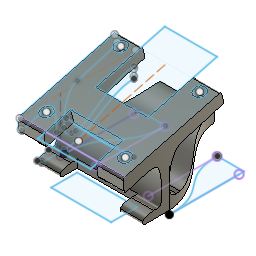
front-short (Autodesk Fusion 360 design; units mm, degrees)
Autodesk Fusion 360 part; units mm, degrees
sketch "Skizze1" plane through (0, 0, 0) normal (1, 0, 0) x (0, 1, 0)
  line L0 (-5, 1) -> (1, 1)
  line L1 (0, 0) -> (0, 14.4867) construction
  line L2 (0, 14.4867) -> (-11.359, 14.4867) construction
  line L3 (0, 14.4867) -> (20, 14.4867) construction
  line L4 (-11.0357, 11.4071) -> (-11.3143, 14.0608)
  line L5 (-10.9451, 14.5964) -> (14.3234, 21.29)
  spline S0 degree 5 poles (1, 1) (1.7814, 1) (3.3248, 1.1441) (5.5821, 1.792) (8.4987, 3.3498) (12.0892, 5.7087) (15.005, 7.2713) (17.261, 7.926) (18.8034, 8.0762) (19.5841, 8.0797) knots 0 0 0 0 0 0 0.2 0.4 0.6 0.8 1 1 1 1 1 1
  line L6 (-1, 1) -> (3, 1)
  line L7 (17.575, 8.0666) -> (21.5749, 8.0843)
  line L8 (20.0592, 10.4933) -> (20.0592, 8.5791)
  arc A0 (20.0592, 10.4933) -> (19.5271, 10.9923) centre (19.5592, 10.4933) ccw
  arc A1 (19.5841, 8.0797) -> (20.0592, 8.5791) centre (19.5592, 8.5791) ccw
  arc A2 (14.9514, 20.8065) -> (14.3234, 21.29) centre (14.4514, 20.8067) ccw
  arc A3 (-11.0357, 11.4071) -> (-10.2738, 11.0351) centre (-10.5384, 11.4593) ccw
  spline S1 degree 5 poles (-10.2738, 11.0351) (-9.3554, 11.3092) (-7.6686, 11.819) (-5.5882, 12.4682) (-3.6466, 13.0308) (-2.2683, 12.9173) (-1.5391, 11.673) (-1.1522, 9.3083) (-0.9068, 6.1018) (-1.0418, 3.5276) (-1.7721, 2.8079) (-2.4824, 3.0034) (-2.8857, 3.1016) (-3.0583, 3.0428) (-3.1208, 2.9828) knots 0 0 0 0 0 0 0.1 0.2 0.3 0.4 0.5 0.6 0.7 0.8 0.9 1 1 1 1 1 1
  line L9 (-14.6982, 9.7143) -> (-5.8494, 12.3559)
  line L10 (-1, 9) -> (-1, 3)
  line L11 (-2.4936, 3.5857) -> (-3.7479, 2.3798)
  spline S2 degree 5 poles (4.5055, 15.1733) (4.1976, 15.0836) (3.6204, 14.8401) (2.8706, 14.2825) (2.0929, 13.1886) (1.4422, 11.4286) (1.0571, 9.5179) (0.8923, 7.6993) (0.918, 6.1755) (1.144, 5.0495) (1.5922, 4.2914) (2.0891, 3.9529) (2.5177, 3.8314) (2.8242, 3.8071) (2.9826, 3.8091) knots 0 0 0 0 0 0 0.1 0.2 0.3 0.4 0.5 0.6 0.7 0.8 0.9 1 1 1 1 1 1
  spline S3 degree 5 poles (19.5271, 10.9923) (18.7621, 10.9405) (17.2555, 10.7096) (15.0658, 9.982) (12.2831, 8.4027) (9.0678, 6.0947) (6.7884, 4.5873) (5.3121, 3.9616) (4.4471, 3.8224) (4.0444, 3.8224) knots 0 0 0 0 0 0 0.2 0.4 0.6 0.8 1 1 1 1 1 1
  line L12 (21.451, 11.1225) -> (17.6033, 10.862)
  line L13 (5.0444, 3.8225) -> (3.0444, 3.8223)
  line L14 (6.7734, 15.8337) -> (2.2376, 14.5129)
  line L15 (0.6508, 8.5379) -> (1.3492, 3.4621)
  line L16 (0.5609, 3.7787) -> (5.4043, 3.8394)
  line L17 (2.9826, 3.8091) -> (4.0444, 3.8224)
  spline S4 degree 5 poles (-5, 1) (-5.1368, 0.9954) (-5.3837, 0.9989) (-5.6734, 1.0427) (-5.921, 1.1673) (-6.0765, 1.3967) (-6.1253, 1.6162) (-6.1334, 1.7945) (-6.1269, 1.9191) (-6.1208, 1.9828) knots 0 0 0 0 0 0 0.2 0.4 0.6 0.8 1 1 1 1 1 1
  spline S5 degree 5 poles (-3.1208, 2.9828) (-3.2537, 2.9767) (-3.5181, 2.9606) (-3.9103, 2.9246) (-4.4234, 2.8514) (-5.0408, 2.697) (-5.5035, 2.4916) (-5.8241, 2.2684) (-6.0241, 2.0839) (-6.1208, 1.9828) knots 0 0 0 0 0 0 0.2 0.4 0.6 0.8 1 1 1 1 1 1
  line L18 (-4.539, 1.0156) -> (-5.461, 0.9844)
  line L19 (-5.8879, 2.2266) -> (-6.3536, 1.7389)
  line L20 (4.5055, 15.1733) -> (15.1184, 18.3262)
  line L21 (15.4586, 18.9363) -> (14.9514, 20.8065)
  arc A4 (15.1184, 18.3262) -> (15.4586, 18.9363) centre (14.976, 18.8055) ccw
  arc A5 (-10.9451, 14.5964) -> (-11.3143, 14.0608) centre (-10.817, 14.113) ccw
  point P0 (-1, 6)
  point P1 (1, 6)
  dimension "d1" = 0.5
  dimension "d2" = 0.5
  dimension "d3" = 0.5
  dimension "d5" = 0.5
  dimension "d24" = 0.5
  dimension "d27" = 0.5
  constraint horizontal L0
  constraint coincident L1.start origin
  constraint perpendicular L0 L1
  constraint perpendicular L1 L2
  constraint perpendicular L1 L3
  constraint midpoint L0.end L6
  constraint vertical L8
  constraint tangent L8 A0
  constraint tangent S0 A1
  constraint tangent L8 A1
  constraint tangent L5 A2
  constraint tangent L4 A3
  constraint midpoint A3.end L9
  constraint midpoint P0 L10
  constraint midpoint S1.end L11
  constraint midpoint A0.end L12
  constraint midpoint S3.end L13
  constraint midpoint S2.start L14
  constraint midpoint P1 L15
  constraint midpoint S2.end L16
  constraint midpoint L0.start L18
  constraint midpoint S4.end L19
  constraint tangent L20 A4
  constraint tangent L21 A4
  constraint coincident L2.end L4
  constraint coincident L2.end L5
  constraint tangent L4 A5
  constraint tangent L5 A5
  measures "d1" radius of A0
  measures "d2" radius of A1
  measures "d3" radius of A2
  measures "d5" radius of A3
  measures "d24" radius of A4
  measures "d27" radius of A5
extrude "Extrusion1" add sketch "Skizze1" along normal blind 28
sketch "Skizze2" plane through (0, -4.3307, 16.3485) normal (0, -0.256068, 0.966659) x (1, 0, 0)
  line L0 (0, 19.2975) -> (0, -6.8425)
  line L1 (28, -6.8425) -> (28, 19.2975)
  line L2 (28, 19.2975) -> (0, 19.2975)
  line L3 (14, -5.0283) -> (14, 19.2975) construction
  line L4 (20.9548, 0) -> (7, 0)
  line L5 (20.9199, 7) -> (7, 7)
  line L6 (20.9199, 7) -> (20.9199, 26)
  line L7 (20.9199, 26) -> (7, 26)
  line L8 (7, 26) -> (7, 7)
  line L9 (7, 0) -> (7, -9)
  line L10 (7, -9) -> (21.0129, -9)
  line L11 (21.0129, -9) -> (20.9548, 0)
  circle A0 centre (3.5, -3) radius 1.5
  circle A1 centre (24.5, -3) radius 1.5
  line L12 (0, -6.8425) -> (28, -6.8425)
  circle A2 centre (3.5, 17.5) radius 1.5
  circle A3 centre (24.5, 17.5) radius 1.5
  dimension "d16" = 3
  dimension "d17" = 3
  dimension "d36" = 3
  dimension "d37" = 3
  constraint midpoint L2 L3.end
  constraint perpendicular L3 L4
  constraint perpendicular L2 L6
  constraint perpendicular L6 L7
  constraint perpendicular L5 L8
  constraint perpendicular L9 L10
  measures "d16" diameter of A0
  measures "d17" diameter of A1
  measures "d36" diameter of A2
  measures "d37" diameter of A3
extrude "Extrusion2" cut sketch "Skizze2" against normal blind 4.5 contours L9 L10 L11 L12 | L4 L9 L11 L12
extrude "Extrusion4" cut sketch "Skizze2" against normal blind 10 contours L2 L6 L7 L8 | L2 L5 L6 L8
sketch "Skizze3" plane through (0, 0, 0) normal (0, 0, 1) x (1, 0, 0)
  line L0 (28, 1) -> (28, 19.5841)
  line L1 (0, 1) -> (0, 19.5841)
  line L2 (7, 20.8024) -> (7, 2.4359)
  line L3 (20.9199, 2.4359) -> (20.9199, 20.8024)
  spline S0 degree 5 poles (28, 1) (28, 2.2287) (27.8554, 4.4703) (27.2053, 7.1862) (25.6424, 9.7666) (23.2775, 12.3598) (21.7146, 14.8926) (21.0645, 17.541) (20.9199, 19.7219) (20.9199, 20.9163) knots 0 0 0 0 0 0 0.2 0.4 0.6 0.8 1 1 1 1 1 1
  line L4 (28, -2) -> (28, 4)
  line L5 (20.9199, 18) -> (20.9199, 23.8326)
  line L6 (20.9199, 20.9163) -> (28, 20.9163)
  line L7 (28, 20.9163) -> (28, 1)
  spline S1 degree 5 poles (0, 1) (0, 2.2274) (0.1429, 4.464) (0.7857, 7.165) (2.3309, 9.716) (4.6691, 12.284) (6.2143, 14.835) (6.8571, 17.536) (7, 19.7726) (7, 21) knots 0 0 0 0 0 0 0.2 0.4 0.6 0.8 1 1 1 1 1 1
  line L8 (0, 1) -> (0, 21)
  line L9 (0, 21) -> (7, 21)
  line L10 (7, 18) -> (7, 24)
  line L11 (0, -2) -> (0, 4)
  line L12 (6, -8.5) -> (6, -1.5706)
  line L13 (6, -1.5706) -> (22, -1.5706)
  line L14 (22, -1.5706) -> (22, -8.5)
  line L15 (22, -8.5) -> (6, -8.5)
  constraint coincident L0.start S0.start
  constraint midpoint L0.start L4
  constraint coincident L0 L4.end
  constraint midpoint S0.end L5
  constraint coincident L3 L5.start
  constraint parallel L3 L5
  constraint perpendicular L5 L6
  constraint coincident L1.start S1.start
  constraint parallel L1 L8
  constraint perpendicular L1 L9
  constraint midpoint S1.end L10
  constraint coincident L2 L10.start
  constraint parallel L2 L10
  constraint midpoint L1.start L11
  constraint coincident L8 L11.end
  constraint vertical L12
  constraint perpendicular L12 L13
  constraint perpendicular L13 L14
  constraint perpendicular L12 L15
extrude "Extrusion5" cut sketch "Skizze3" along normal blind 11 contours L0 S0 L4 L5 L6 L7
extrude "Extrusion6" cut sketch "Skizze2" against normal blind 4 contours A0 | A1
extrude "Extrusion7" cut sketch "Skizze3" along normal blind 4 contours L12 L13 L14 L15
extrude "Extrusion14" cut sketch "Skizze2" against normal blind 2.5 contours A2 | A3
ref_plane "Arbeitsebene2" through (13.9774, -3.8698, 14.6086) normal (0, -0.966659, -0.256068) x (-1, 0, 0)
sketch "Skizze7" plane through (13.9774, -3.8698, 14.6086) normal (0, -0.966659, -0.256068) x (-1, 0, 0)
  spline S0 degree 5 poles (9.026, 1.6628) (8.2399, 1.8098) (6.7, 2.0711) (4.4872, 2.3644) (1.6929, 2.5775) (-1.705, 2.5877) (-4.492, 2.3838) (-6.6945, 2.0861) (-8.2251, 1.8159) (-9.0059, 1.6628) knots 0 0 0 0 0 0 0.2 0.4 0.6 0.8 1 1 1 1 1 1
  line L0 (11.0137, 1.291) -> (7.0384, 2.0346)
  line L1 (-7.0331, 2.0496) -> (-10.9787, 1.276)
  line L2 (9.026, 1.6628) -> (-9.0059, 1.6628)
  constraint midpoint S0.start L0
  constraint midpoint S0.end L1
  constraint horizontal L2
extrude "Extrusion15" cut sketch "Skizze7" along normal blind 8
extrude "Extrusion16" cut sketch "Skizze7" against normal blind 20.5
extrude "Extrusion17" cut sketch "Skizze3" along normal blind 12 contours L1 S1 L8 L9 L10 L11
